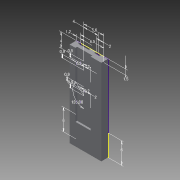
# Autodesk Inventor part: key
Saved by Autodesk Inventor 2013 (Build 170138000, 138)
## iProperties
Created: 2014-05-15
Part Number: key
Material: 一般
Document SubType Name: Modeling
Designer: andou
Density: 1 g/cm^3
Author: andou
Autodesk Inventor part; units mm, degrees
ref_plane "YZ Plane" through (0, 0, 0) normal (1, 0, 0) x (0, 1, 0)
ref_plane "XZ Plane" through (0, 0, 0) normal (0, 1, 0) x (-1, 0, 0)
ref_plane "XY Plane" through (0, 0, 0) normal (0, 0, 1) x (1, 0, 0)
sketch "スケッチ1" plane through (0, 0, 0) normal (0, 1, 0) x (-1, 0, 0)
  line L0 (-4.45, 12) -> (4.45, 12)
  line L1 (4.45, 12) -> (4.45, -12)
  line L2 (4.45, -12) -> (-4.45, -12)
  line L3 (-4.45, -12) -> (-4.45, 12)
  point P0 (0, 0)
  dimension "d0" = 8.9
  dimension "d2" = 24
  dimension "d3" = 4.45
  dimension "d4" = 12
  constraints: 8 end point, 2 parallel, 1 horizontal, 1 perpendicular
  measures "d0" distance of L0.start L0.end
  measures "d2" distance of L2.end L0.start
  measures "d3" distance from line of point (0, 0) L3
  measures "d4" distance from line of point (0, 0) L0
extrude "押し出し1" add sketch "スケッチ1" along normal blind 1.9
sketch "スケッチ2" plane through (0, 1.9, 0) normal (0, 1, 0) x (1, 0, 0)
  line L0 (-4.45, -12) -> (4.45, -12) projected
  line L1 (4.45, -12) -> (4.45, 12) projected
  line L2 (4.45, 12) -> (-4.45, 12) projected
  line L3 (-4.45, 12) -> (-4.45, -12) projected
  line L4 (-4.45, -12) -> (-3.25, -12)
  line L5 (-3.25, -12) -> (-3.25, 6)
  line L6 (-3.25, 6) -> (-4.45, 6)
  line L7 (-4.45, 6) -> (-4.45, -12)
  line L8 (4.45, -12) -> (3.25, -12)
  line L9 (3.25, -12) -> (3.25, 6)
  line L10 (3.25, 6) -> (4.45, 6)
  line L11 (4.45, 6) -> (4.45, -12)
  line L12 (1.25, -12) -> (3.25, -10.5)
  line L13 (-2.35, -12) -> (-2.35, 6)
  line L14 (-2.35, 6) -> (-3.25, 6)
  line L15 (1.65, -12) -> (-2.35, -8)
  line L16 (-2.35, -7.1) -> (-2.15, -6.9)
  line L17 (-2.15, -6.9) -> (-2.35, -6.7)
  line L18 (-2.35, -5.8) -> (-0.35, -3.8)
  line L19 (-0.35, -3.8) -> (-2.35, -1.8)
  line L20 (-2.35, -0.9) -> (-2.15, -0.7)
  line L21 (-2.15, -0.7) -> (-2.35, -0.5)
  line L22 (-2.35, 0.4) -> (-0.35, 2.4)
  line L23 (-0.35, 2.4) -> (-3.25, 5.3)
  point P0 (0, 0)
  dimension "d7" = 6.5
  dimension "d9" = 1.2
  dimension "d10" = 6
  dimension "d11" = 6
  dimension "d12" = 1.5
  dimension "d13" = 2
  dimension "d20" = 5.6
  dimension "d22" = 4
  dimension "d23" = 4
  dimension "d24" = 0.2
  dimension "d25" = 0.9
  dimension "d26" = 0.9
  dimension "d27" = 2
  dimension "d28" = 0.2
  dimension "d29" = 0.9
  dimension "d30" = 2
  dimension "d31" = 0.9
  dimension "d32" = 135
  constraints: 38 end point, 9 perpendicular, 5 point on line, 4 parallel, 3 horizontal, 1 vertical, 11 other
  measures "d7" distance between parallel lines of L9 L5
  measures "d9" distance between parallel lines of L3 L5
  measures "d10" distance between parallel lines of L2 L6
  measures "d11" distance between parallel lines of L2 L10
  measures "d12" vertical distance of L12.start L12.end
  measures "d13" horizontal distance of L12.start L12.end
  measures "d22" horizontal distance of L15.start L15.end
  measures "d23" horizontal distance of L15.start L15.end
  measures "d25" distance of L15.end L16.start
  measures "d26" distance of L17.end L18.start
  measures "d27" horizontal distance of L18.start L18.end
  measures "d28" horizontal distance of L20.start L20.end
  measures "d29" distance of L19.end L20.start
  measures "d30" horizontal distance of L22.start L22.end
  measures "d31" distance of L21.end L22.start
  measures "d32" angle to the sketch x axis of L22
sketch "スケッチ3" plane through (0, 1.9, 0) normal (0, 1, 0) x (1, 0, 0)
  line L0 (-4.45, -12) -> (4.45, -12) projected
  line L1 (4.45, 12) -> (-4.45, 12) projected
  line L2 (-4.45, 12) -> (-4.45, -12) projected
  line L3 (-3.45, -12) -> (-0.45, -12)
  line L4 (-0.45, -12) -> (-0.45, 12)
  line L5 (-0.45, 12) -> (-3.45, 12)
  line L6 (-3.45, 12) -> (-3.45, -12)
  line L7 (1.05, 12) -> (2.55, 12)
  line L8 (2.55, 12) -> (2.55, -12)
  line L9 (2.55, -12) -> (1.05, -12)
  line L10 (1.05, -12) -> (1.05, 12)
  point P0 (0, 0)
  dimension "d35" = 1
  dimension "d36" = 3
  dimension "d37" = 1.5
  dimension "d38" = 1.5
  constraints: 16 end point, 4 parallel, 4 point on line, 2 horizontal, 2 perpendicular
  measures "d35" distance between parallel lines of L2 L6
  measures "d36" distance between parallel lines of L6 L4
  measures "d37" distance between parallel lines of L4 L10
  measures "d38" distance between parallel lines of L8 L10
sketch "スケッチ4" plane through (0, 0, 0) normal (0, -1, 0) x (1, 0, 0)
  line L0 (4.45, 12) -> (-4.45, 12) projected
  line L1 (-4.45, -12) -> (4.45, -12) projected
  line L2 (4.45, -12) -> (4.45, 12) projected
  line L3 (-2.8, 12) -> (1.45, 12)
  line L4 (1.45, 12) -> (1.45, -6)
  line L5 (1.45, -6) -> (-2.8, -6)
  line L6 (-2.8, -6) -> (-2.8, 12)
  point P0 (0, 0)
  dimension "d39" = 6
  dimension "d40" = 4.25
  dimension "d41" = 3
  constraints: 8 end point, 2 parallel, 1 horizontal, 1 perpendicular, 1 point on line
  measures "d39" distance between parallel lines of L5 L1
  measures "d40" distance between parallel lines of L4 L6
  measures "d41" distance between parallel lines of L2 L4
extrude "押し出し3" cut sketch "スケッチ4" against normal blind 0.5
extrude "押し出し4" cut sketch "スケッチ3" against normal blind 0.5 contours L6 L1 L4 L0 | L10 L1 L8 L0
